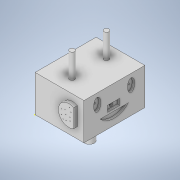
# Autodesk Inventor part: head part 2
Saved by Autodesk Inventor 2021 (Build 250183000, 183)
## iProperties
Created: 2021-07-09
Part Number: head part 2
Material: Generic
Document SubType Name: Modeling
Designer: V Hoskoti
Density: 1 g/cm^3
Appearance: Default
Author: V Hoskoti
Autodesk Inventor part; units mm, degrees
ref_plane "YZ Plane" through (0, 0, 0) normal (1, 0, 0) x (0, 1, 0)
ref_plane "XZ Plane" through (0, 0, 0) normal (0, 1, 0) x (-1, 0, 0)
ref_plane "XY Plane" through (0, 0, 0) normal (0, 0, 1) x (1, 0, 0)
sketch "Sketch1" plane through (0, 0, 0) normal (0, 0, 1) x (1, 0, 0)
  line L0 (0, 0) -> (250, 0)
  line L1 (250, 0) -> (250, 150)
  line L2 (250, 150) -> (0, 150)
  line L3 (0, 150) -> (0, 0)
  ellipse E0 centre (61.2005, 103.0437) end of major axis (61.2005, 79.9077) minor radius 20.4496
  ellipse E1 centre (186.6962, 103.0437) end of major axis (186.6962, 79.9077) minor radius 20.4496
  arc A0 (59.086, 49.2762) -> (190.914, 49.2762) centre (125, 119.8778) ccw
  line L4 (59.086, 49.2762) -> (190.914, 49.2762)
  constraints: 10 end point, 3 centre point, 3 horizontal, 2 point on circle, 1 perpendicular, 1 vertical, 2 other
extrude "Extrusion1" add sketch "Sketch1" along normal blind 200 contours L3 L2 L1 L0 | E0 | E1 | L4 A0
sketch "Sketch2" plane through (0, 0, 0) normal (0, 0, -1) x (-1, 0, 0)
  point P0 (0, 0)
sketch "Sketch3" plane through (0, 0, 200) normal (0, 0, 1) x (1, 0, 0)
  ellipse E0 centre (54.3866, 108.1481) end of major axis (54.3866, 81.8925) minor radius 14.5317
  ellipse E1 centre (193.1662, 108.1481) end of major axis (193.1662, 81.8925) minor radius 14.5317
  arc A0 (66.4831, 50.9455) -> (182.3199, 50.9455) centre (124.4015, 103.7721) ccw
  line L0 (66.4831, 50.9455) -> (182.3199, 50.9455)
  point P0 (0, 0)
  constraints: 3 centre point, 2 end point, 2 point on circle, 1 horizontal, 2 other
extrude "Extrusion2" cut sketch "Sketch3" against normal blind 10 contours E0
extrude "Extrusion3" cut sketch "Sketch3" against normal blind 10 contours E1
extrude "Extrusion4" cut sketch "Sketch3" against normal blind 10 contours L0 A0
sketch "Sketch4" plane through (250, 0, 0) normal (1, 0, 0) x (0, 0, -1)
  arc A0 (-152.7748, 40.0737) -> (-152.7748, 122.4086) centre (-136.5666, 81.2411) ccw
  line L0 (-152.7748, 40.0737) -> (-152.7748, 122.4086)
  point P0 (0, 0)
  constraints: 2 end point, 2 point on circle, 1 centre point, 1 vertical
extrude "Extrusion5" add sketch "Sketch4" along normal blind 15
sketch "Sketch5" plane through (0, 0, 0) normal (-1, 0, 0) x (0, 0, 1)
  line L0 (152.7748, 40.0737) -> (152.7748, 122.4086) projected
  arc A0 (173.1982, 118.4375) -> (173.1982, 44.0448) centre (152.7748, 81.2411) ccw
  line L1 (173.1982, 118.4375) -> (173.1982, 44.0448)
  point P0 (0, 0)
  constraints: 2 end point, 2 point on circle, 1 centre point, 1 midpoint, 1 vertical
extrude "Extrusion6" add sketch "Sketch5" along normal blind 15
sketch "Sketch6" plane through (0, 150, 0) normal (0, 1, 0) x (1, 0, 0)
  circle A0 centre (54.7125, -97.0495) radius 10
  circle A1 centre (195.4016, -97.0495) radius 10
  point P0 (0, 0)
  dimension "d14" = 20
  dimension "d15" = 20
  constraints: 2 centre point
  measures "d14" diameter of A0
  measures "d15" diameter of A1
extrude "Extrusion7" add sketch "Sketch6" along normal blind 100 contours A0
extrude "Extrusion8" add sketch "Sketch6" along normal blind 100 contours A1
sketch "Sketch7" plane through (0, 0, 0) normal (0, -1, 0) x (1, 0, 0)
  point P0 (0, 0)
sketch "Sketch9" plane through (0, 0, 0) normal (0, -1, 0) x (1, 0, 0)
  circle A0 centre (120.0971, 102.6638) radius 20
  point P0 (0, 0)
  dimension "d20" = 40
  constraints: 1 centre point
  measures "d20" diameter of A0
extrude "Extrusion9" add sketch "Sketch9" along normal blind 100
sketch "Sketch10" plane through (-15, 0, 0) normal (-1, 0, 0) x (0, 0, 1)
  point P0 (0, 0)
  point P1 (140.6371, 77.6587)
hole "Hole1" at (-15, 77.6587, 140.6371) direction (1, 0, 0) diameter 2 depth 5 tip angle 118
sketch "Sketch11" plane through (-15, 0, 0) normal (-1, 0, 0) x (0, 0, 1)
  point P0 (0, 0)
  point P1 (137.5819, 94.0305)
hole "Hole2" at (-15, 94.0305, 137.5819) direction (1, 0, 0) diameter 2 depth 5 tip angle 118
sketch "Sketch12" plane through (-15, 0, 0) normal (-1, 0, 0) x (0, 0, 1)
  point P0 (0, 0)
  point P1 (161.7546, 97.274)
hole "Hole3" at (-15, 97.274, 161.7546) direction (1, 0, 0) diameter 2 depth 5 tip angle 118
sketch "Sketch13" plane through (-15, 0, 0) normal (-1, 0, 0) x (0, 0, 1)
  point P0 (0, 0)
  point P1 (122.1615, 69.1759)
hole "Hole4" at (-15, 69.1759, 122.1615) direction (1, 0, 0) diameter 2 depth 5 tip angle 118
sketch "Sketch14" plane through (-15, 0, 0) normal (-1, 0, 0) x (0, 0, 1)
  point P0 (0, 0)
  point P1 (142.1664, 58.2443)
hole "Hole5" at (-15, 58.2443, 142.1664) direction (1, 0, 0) diameter 2 depth 5 tip angle 118
sketch "Sketch15" plane through (-15, 0, 0) normal (-1, 0, 0) x (0, 0, 1)
  point P0 (0, 0)
  point P1 (154.8779, 110.2581)
hole "Hole6" at (-15, 110.2581, 154.8779) direction (1, 0, 0) diameter 2 depth 5 tip angle 118
sketch "Sketch16" plane through (-15, 0, 0) normal (-1, 0, 0) x (0, 0, 1)
  point P0 (0, 0)
  point P1 (158.2121, 63.5601)
hole "Hole7" at (-15, 63.5601, 158.2121) direction (1, 0, 0) diameter 2 depth 5 tip angle 118
sketch "Sketch17" plane through (-15, 0, 0) normal (-1, 0, 0) x (0, 0, 1)
  point P0 (0, 0)
  point P1 (157.5869, 77.3239)
hole "Hole8" at (-15, 77.3239, 157.5869) direction (1, 0, 0) diameter 2 depth 5 tip angle 118
sketch "Sketch18" plane through (-15, 0, 0) normal (-1, 0, 0) x (0, 0, 1)
  point P0 (0, 0)
  point P1 (122.5782, 89.2357)
hole "Hole9" at (-15, 89.2357, 122.5782) direction (1, 0, 0) diameter 2 depth 5 tip angle 118
sketch "Sketch19" plane through (-15, 0, 0) normal (-1, 0, 0) x (0, 0, 1)
  point P0 (0, 0)
  point P1 (130.0801, 56.8932)
hole "Hole10" at (-15, 56.8932, 130.0801) direction (1, 0, 0) diameter 2 depth 5 tip angle 118
sketch "Sketch20" plane through (265, 0, 0) normal (1, 0, 0) x (0, 0, -1)
  point P0 (0, 0)
  point P1 (-130.0065, 99.3663)
hole "Hole11" at (265, 99.3663, 130.0065) direction (-1, 0, 0) diameter 2 depth 5 tip angle 118
sketch "Sketch21" plane through (265, 0, 0) normal (1, 0, 0) x (0, 0, -1)
  point P0 (0, 0)
  point P1 (-115.2751, 85.4238)
hole "Hole12" at (265, 85.4238, 115.2751) direction (-1, 0, 0) diameter 2 depth 5 tip angle 118
sketch "Sketch22" plane through (265, 0, 0) normal (1, 0, 0) x (0, 0, -1)
  point P0 (0, 0)
  point P1 (-139.5268, 76.7471)
hole "Hole13" at (265, 76.7471, 139.5268) direction (-1, 0, 0) diameter 2 depth 5 tip angle 118
sketch "Sketch23" plane through (265, 0, 0) normal (1, 0, 0) x (0, 0, -1)
  point P0 (0, 0)
  point P1 (-117.355, 66.6893)
hole "Hole14" at (265, 66.6893, 117.355) direction (-1, 0, 0) diameter 2 depth 5 tip angle 118
sketch "Sketch24" plane through (265, 0, 0) normal (1, 0, 0) x (0, 0, -1)
  point P0 (0, 0)
  point P1 (-117.0358, 98.3789)
hole "Hole15" at (265, 98.3789, 117.0358) direction (-1, 0, 0) diameter 2 depth 5 tip angle 118
sketch "Sketch25" plane through (265, 0, 0) normal (1, 0, 0) x (0, 0, -1)
  point P0 (0, 0)
  point P1 (-134.2147, 59.0465)
hole "Hole16" at (265, 59.0465, 134.2147) direction (-1, 0, 0) diameter 2 depth 5 tip angle 118
sketch "Sketch26" plane through (265, 0, 0) normal (1, 0, 0) x (0, 0, -1)
  point P0 (0, 0)
  point P1 (-127.1753, 78.1775)
hole "Hole17" at (265, 78.1775, 127.1753) direction (-1, 0, 0) diameter 2 depth 5 tip angle 118
sketch "Sketch27" plane through (265, 0, 0) normal (1, 0, 0) x (0, 0, -1)
  point P0 (0, 0)
  point P1 (-141.5728, 92.3364)
hole "Hole18" at (265, 92.3364, 141.5728) direction (-1, 0, 0) diameter 2 depth 5 tip angle 118
sketch "Sketch28" plane through (265, 0, 0) normal (1, 0, 0) x (0, 0, -1)
  point P0 (0, 0)
  point P1 (-133.6045, 107.8408)
hole "Hole19" at (265, 107.8408, 133.6045) direction (-1, 0, 0) diameter 2 depth 5 tip angle 118
sketch "Sketch29" plane through (0, 0, 200) normal (0, 0, 1) x (1, 0, 0)
  line L0 (96.2975, 84.9409) -> (146.2975, 84.9409)
  line L1 (146.2975, 84.9409) -> (146.2975, 59.9409)
  line L2 (146.2975, 59.9409) -> (96.2975, 59.9409)
  line L3 (96.2975, 59.9409) -> (96.2975, 84.9409)
  point P0 (0, 0)
  dimension "d156" = 50
  dimension "d157" = 25
  constraints: 8 end point, 2 parallel, 1 horizontal, 1 perpendicular
  measures "d156" distance of L1.end L2.end
  measures "d157" distance of L0.end L1.end
extrude "Extrusion10" cut sketch "Sketch29" against normal blind 10
sketch "Sketch30" plane through (0, 0, 190) normal (0, 0, 1) x (1, 0, 0)
  circle A0 centre (121.2975, 71.6727) radius 7.5
  point P0 (0, 0)
  dimension "d160" = 15
  constraints: 1 centre point
  measures "d160" diameter of A0
extrude "Extrusion11" cut sketch "Sketch30" against normal blind 50
sketch "Sketch31" plane through (0, 0, 190) normal (0, 0, 1) x (1, 0, 0)
  point P0 (0, 0)
  point P1 (54.4067, 107.7576)
hole "Hole20" at (54.4067, 107.7576, 190) direction (0, 0, -1) diameter 5 depth 5 tip angle 118
sketch "Sketch32" plane through (0, 0, 190) normal (0, 0, 1) x (1, 0, 0)
  point P0 (0, 0)
  point P1 (195.0454, 105.5749)
hole "Hole21" at (195.0454, 105.5749, 190) direction (0, 0, -1) diameter 5 depth 5 tip angle 118
body "Solid1"
